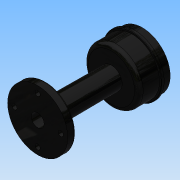
# Autodesk Inventor part: Signal_tower_A
Saved by Autodesk Inventor 2017.3 (Build 213256000, 256)
## iProperties
Created: 2017-03-21
Part Number: Signal_tower_A
Material: PC/ABS plast
Document SubType Name: Modeling
Mass: 62.2783 g
Surface Area: 348.774 cm^2
Volume: 174.316 cm^3
Density: 0.357273 g/cm^3
Appearance: Železo – černá
Stock Number: SIEMENS
Hmotnost: 0
Hotovo: 0
Objem: 0
X: 0
Y: 0
Z: 0
Author: CAD
Autodesk Inventor part; units mm, degrees
ref_plane "YZ Plane" through (0, 0, 0) normal (1, 0, 0) x (0, 1, 0)
ref_plane "XZ Plane" through (0, 0, 0) normal (0, 1, 0) x (-1, 0, 0)
ref_plane "XY Plane" through (0, 0, 0) normal (0, 0, 1) x (1, 0, 0)
sketch "Náčrt2" plane through (0, 0, 0) normal (0, 0, 1) x (1, 0, 0)
  line L0 (-7.5, 0) -> (-35, 0)
  line L1 (-35, 0) -> (-35, 7.4035)
  line L2 (-33.4432, 9.3538) -> (-16.0914, 13.2974)
  line L3 (0, 0) -> (0, 103.3907) construction
  line L4 (-12.978, 17.1702) -> (-12.5, 86)
  line L5 (-12.5, 86) -> (-27, 86)
  line L6 (-32, 91) -> (-32, 110)
  arc A0 (-32, 91) -> (-27, 86) centre (-27, 91) ccw
  line L7 (-27, 0) -> (-27, 15.9708)
  line L8 (-27, 15.9708) -> (-32.5, 15.9708)
  line L9 (-32.5, 15.9708) -> (-32.5, 6)
  line L10 (-32.5, 6) -> (-30, 6)
  line L11 (-30, 6) -> (-30, 0)
  arc A1 (-33.4432, 9.3538) -> (-35, 7.4035) centre (-33, 7.4035) ccw
  arc A2 (-16.0914, 13.2974) -> (-12.978, 17.1702) centre (-16.9779, 17.1979) ccw
  line L12 (-32, 110) -> (-34.5, 110)
  line L13 (-34.5, 110) -> (-34.5, 113)
  line L14 (-34.5, 113) -> (-32.5, 113)
  line L15 (-32.5, 113) -> (-32.5, 122)
  line L16 (-32.5, 122) -> (-7.5, 122)
  line L17 (-7.5, 122) -> (-7.5, 0)
  line L18 (-7.5, 0) -> (0, 0) construction
  point P0 (-35, 9)
  point P1 (-13, 14)
  dimension "d0" = 70
  dimension "d1" = 9
  dimension "d2" = 14
  dimension "d4" = 26
  dimension "d5" = 25
  dimension "d6" = 64
  dimension "d7" = 5
  dimension "d8" = 86
  dimension "d9" = 27
  dimension "d10" = 6
  dimension "d11" = 11
  dimension "d12" = 6
  dimension "d13" = 2
  dimension "d14" = 4
  dimension "d15" = 15
  dimension "d16" = 24
  dimension "d17" = 69
  dimension "d18" = 65
  dimension "d19" = 27
  dimension "d20" = 36
  dimension "d26" = 9
  dimension "d27" = 3
  constraints: 38 end point, 11 perpendicular, 6 point on circle, 6 point on line, 6 tangent, 4 horizontal, 3 centre point, 1 vertical
  measures "d0" diameter of L1 L3
  measures "d1" distance of L0.end point (-35, 9)
  measures "d2" distance from line of point (-13, 14) L0
  measures "d4" diameter of point (-13, 14) L3
  measures "d5" diameter of L4.end L3
  measures "d6" diameter of L6 L3
  measures "d7" radius of A0
  measures "d8" distance between parallel lines of L5 L0
  measures "d9" distance of L3.start L7.start
  measures "d10" diameter of L11 L7
  measures "d11" diameter of L9 L7
  measures "d12" distance between parallel lines of L10 L0
  measures "d13" radius of A1
  measures "d14" radius of A2
  measures "d15" diameter of L17 L3
  measures "d16" distance between parallel lines of L12 L5
  measures "d17" diameter of L13 L3
  measures "d18" diameter of L15 L3
  measures "d19" distance between parallel lines of L14 L5
  measures "d20" distance between parallel lines of L5 L16
  measures "d26" distance between parallel lines of L14 L16
  measures "d27" distance between parallel lines of L12 L14
revolve "Rotace1" add sketch "Náčrt2" angle 360 about axis through (0, 0, 0) along (0, 1, 0) contours L0 L7 L2 A2 L4 L5 A0 L6 L12 L13 L14 L15 L16 L17 | L0 L11 L10 L9 L2 L7 | L0 L1 A1 L2 L9 L10 L11
revolve "Rotace2" cut sketch "Náčrt2" angle 360 about axis through (-27, 0, 0) along (0, 1, 0) contours L0 L11 L10 L9 L2 L7 | L2 L9 L8 L7
pattern_circular "Kruhové pole1" count 4 over 360 about axis through (0, -10, 0) along (0, 1, 0) of "Rotace2"
chamfer "Zkosení1" distance 0.5 angle 45 1 edges at (34.5, 110, 0)
